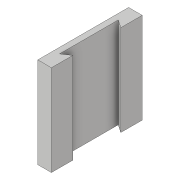
# Autodesk Inventor part: Sliding lock female test
Saved by Autodesk Inventor 2019 (Build 230136000, 136)
## iProperties
Created: 2019-10-09
Part Number: Sliding lock female test
Material: Generic
Document SubType Name: Modeling
Designer: ball
Density: 1 g/cm^3
Appearance: Default
Author: ball
Autodesk Inventor part; units mm, degrees
ref_plane "YZ Plane" through (0, 0, 0) normal (1, 0, 0) x (0, 1, 0)
ref_plane "XZ Plane" through (0, 0, 0) normal (0, 1, 0) x (-1, 0, 0)
ref_plane "XY Plane" through (0, 0, 0) normal (0, 0, 1) x (1, 0, 0)
sketch "Sketch1" plane through (0, 0, 0) normal (0, 1, 0) x (-1, 0, 0)
  line L0 (0, 0) -> (-3.81, 0)
  line L1 (-3.81, -25.4) -> (0, -25.4)
  line L2 (0, -25.4) -> (0, 0)
  line L3 (-3.81, -6.35) -> (-1.905, -6.35) construction
  line L4 (-1.905, -6.35) -> (-1.905, -19.05) construction
  line L5 (-1.905, -19.05) -> (-3.81, -19.05) construction
  line L6 (-1.905, -6.35) -> (-1.905, -5.08) construction
  line L7 (-1.905, -5.08) -> (-3.81, -6.35) construction
  line L8 (-1.905, -19.05) -> (-1.905, -20.32) construction
  line L9 (-1.905, -20.32) -> (-3.81, -19.05) construction
  line L10 (-1.5875, -4.4867) -> (-1.5875, -6.35)
  line L11 (-1.5875, -6.35) -> (-1.5875, -19.05)
  line L12 (-1.5875, -19.05) -> (-1.5875, -20.9133)
  line L13 (-1.5875, -20.9133) -> (-3.81, -19.4316)
  line L14 (-3.81, -5.9684) -> (-1.5875, -4.4867)
  line L15 (-3.81, 0) -> (-3.81, -5.9684)
  line L16 (-3.81, -19.4316) -> (-3.81, -25.4)
  dimension "d0" = 3.81
  dimension "d1" = 25.4
  dimension "d3" = 12.7
  dimension "d4" = 6.35
  dimension "d5" = 1.27
  dimension "d6" = 1.27
  dimension "d7" = 0.3175
  constraints: 34 end point, 4 parallel, 3 perpendicular, 2 horizontal, 2 vertical, 2 other
  measures "d0" distance of L1.end L1.start
  measures "d1" distance of L1.start L0.end
  measures "d3" distance of L3.end L4.end
  measures "d4" distance between parallel lines of L3 L0
  measures "d5" distance of L3.end L6.end
  measures "d6" distance of L4.end L8.end
  measures "d7" distance between parallel lines of L6 L10
extrude "Extrusion1" add sketch "Sketch1" along normal blind 25.4
body "Solid1"
